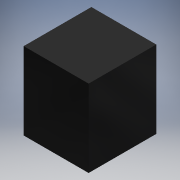
# Autodesk Inventor part: KS diant C
Saved by Autodesk Inventor 2019 (Build 230136000, 136)
## iProperties
Created: 2020-06-04
Part Number: KS diant C
Material: Plástico, preto opaco
Document SubType Name: Modeling
Designer: eliane
Density: 0.952 g/cm^3
Appearance: Liso - Preto
Author: eliane
Autodesk Inventor part; units mm, degrees
ref_plane "YZ Plane" through (0, 0, 0) normal (1, 0, 0) x (0, 1, 0)
ref_plane "XZ Plane" through (0, 0, 0) normal (0, 1, 0) x (-1, 0, 0)
ref_plane "XY Plane" through (0, 0, 0) normal (0, 0, 1) x (1, 0, 0)
sketch "Esboço1" plane through (0, 0, 0) normal (0, 0, 1) x (1, 0, 0)
  line L0 (0, 0) -> (44, 0)
  line L1 (44, 0) -> (44, 50)
  line L2 (44, 50) -> (0, 50)
  line L3 (0, 50) -> (0, 0)
  dimension "d0" = 44
  dimension "d1" = 50
  constraints: 8 end point, 2 parallel, 1 horizontal, 1 perpendicular
  measures "d0" distance of L2.end L1.end
  measures "d1" distance of L1.end L0.end
extrude "Extrusão1" add sketch "Esboço1" along normal blind 3
sketch "Esboço2" plane through (0, 0, 0) normal (-1, 0, 0) x (0, 0, 1)
  line L0 (0, 0) -> (0, 50) projected
  line L1 (0, 50) -> (-16, 50)
  line L2 (-16, 50) -> (-16, 0)
  line L3 (-16, 0) -> (0, 0)
  line L4 (0, 0) -> (0, 50)
  line L5 (0, 50) -> (-8, 50) construction
  line L6 (-8, 50) -> (-8, 42) construction
  line L7 (0, 0) -> (-8, 0) construction
  line L8 (-8, 0) -> (-8, 8) construction
  circle A0 centre (-8, 42) radius 3
  circle A1 centre (-8, 8) radius 3
  dimension "d4" = 16
  dimension "d5" = 50
  dimension "d6" = 8
  dimension "d7" = 8
  dimension "d8" = 8
  dimension "d9" = 8
  dimension "d10" = 6
  dimension "d11" = 6
  constraints: 16 end point, 3 perpendicular, 2 centre point, 2 coincident, 2 midpoint, 2 parallel, 1 horizontal
  measures "d4" distance of L3.end L2.end
  measures "d5" distance of L2.end L1.end
  measures "d6" distance of L0.end L5.end
  measures "d7" distance of L5.end L6.end
  measures "d8" distance of L3.end L7.end
  measures "d9" distance of L7.end L8.end
  measures "d10" diameter of A0
  measures "d11" diameter of A1
extrude "Extrusão2" add sketch "Esboço2" against normal blind 3
sketch "Esboço3" plane through (44, 0, 0) normal (1, 0, 0) x (0, 0, -1)
  line L0 (0, 50) -> (-3, 50) projected
  line L1 (-3, 50) -> (46, 50)
  line L2 (46, 50) -> (46, 0)
  line L3 (46, 0) -> (-3, 0)
  line L4 (-3, 0) -> (-3, 50)
  point P0 (0, 0)
  dimension "d14" = 49
  constraints: 8 end point, 2 parallel, 1 horizontal, 1 perpendicular
  measures "d14" distance of L2.end L3.end
extrude "Extrusão3" add sketch "Esboço3" along normal blind 3
sketch "Esboço4" plane through (44, 0, -46) normal (0, 0, -1) x (-1, 0, 0)
  line L0 (0, 50) -> (41, 50) construction
  line L1 (0, 50) -> (8, 50) construction
  line L2 (8, 50) -> (8, 42) construction
  line L3 (0, 50) -> (0, 0) construction
  line L4 (0, 0) -> (8, 0) construction
  line L5 (41, 0) -> (0, 0) construction
  line L6 (8, 0) -> (8, 8) construction
  circle A0 centre (8, 42) radius 3
  circle A1 centre (8, 8) radius 3
  line L7 (0, 50) -> (16, 50)
  line L8 (16, 50) -> (16, 42)
  line L9 (16, 42) -> (11, 35.755)
  line L10 (11, 35.755) -> (0, 35.755)
  line L11 (0, 50) -> (0, 35.755)
  line L12 (0, 0) -> (16, 0)
  line L13 (16, 0) -> (16, 8)
  line L14 (16, 8) -> (11, 14.245)
  line L15 (11, 14.245) -> (0, 14.245)
  line L16 (0, 0) -> (0, 14.245)
  point P0 (44, 0)
  dimension "d17" = 8
  dimension "d18" = 8
  dimension "d19" = 8
  dimension "d20" = 8
  dimension "d21" = 6
  dimension "d22" = 6
  dimension "d23" = 16
  dimension "d24" = 8
  dimension "d25" = 8
  dimension "d26" = 8
  constraints: 28 end point, 6 perpendicular, 6 point on line, 2 centre point, 2 coincident, 1 collinear, 1 vertical
  measures "d17" distance of L0.start L1.end
  measures "d18" distance of L1.end L2.end
  measures "d19" distance of L3.end L4.end
  measures "d20" distance of L4.end L6.end
  measures "d21" diameter of A0
  measures "d22" diameter of A1
  measures "d23" distance of L0.start L7.end
  measures "d24" distance of L7.end L8.end
  measures "d25" distance of L8.end L9.end
  measures "d26" distance of L13.end L14.end
extrude "Extrusão4" add sketch "Esboço4" against normal blind 3
sketch "Esboço5" plane through (0, 50, -16) normal (0, 1, 0) x (1, 0, 0)
  line L0 (0, 0) -> (0, -19) projected
  line L1 (47, 30) -> (47, -19) projected
  line L2 (0, -19) -> (47, -19)
  line L3 (47, -19) -> (47, 30)
  line L4 (47, 30) -> (0, 30)
  line L5 (0, 30) -> (0, -19)
  point P0 (0, -16)
  constraints: 8 end point, 2 parallel, 1 horizontal, 1 perpendicular
extrude "Extrusão5" add sketch "Esboço5" along normal blind 3
sketch "Esboço6" plane through (0, 0, -16) normal (0, -1, 0) x (1, 0, 0)
  line L0 (47, -30) -> (0, -30) projected
  line L1 (0, 19) -> (47, 19) projected
  line L2 (0, -30) -> (47, -30)
  line L3 (47, -30) -> (47, 19)
  line L4 (47, 19) -> (0, 19)
  line L5 (0, 19) -> (0, -30)
  point P0 (0, 16)
  constraints: 8 end point, 2 parallel, 1 horizontal, 1 perpendicular
extrude "Extrusão6" add sketch "Esboço6" along normal blind 3
sketch "Esboço7" plane through (0, -3, -16) normal (0, -1, 0) x (1, 0, 0)
  point P0 (0, 16)
  point P1 (5.9184, 10.7829)
  point P2 (9.9362, 10.9743)
hole "Furo1" at (5.9184, -3, -5.2171) at (9.9362, -3, -5.0257) direction (0, 1, 0) diameter 2 depth 3 tip angle 118
sketch "Esboço8" plane through (0, -3, -16) normal (0, -1, 0) x (1, 0, 0)
  circle A0 centre (5.9184, 10.7829) radius 1 projected
sketch "Esboço9" plane through (0, -3, -16) normal (0, -1, 0) x (1, 0, 0)
  circle A0 centre (9.9362, 10.9743) radius 1 projected
